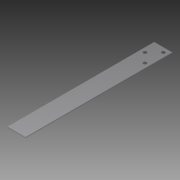
# Autodesk Inventor part: big ball holder_MIR
Saved by Autodesk Inventor 2014 SP1 (Build 180222100, 222)
## iProperties
Created: 2013-11-15
Part Number: big ball holder_MIR
Material: Polycarbonate, Clear
Document SubType Name: Modeling
Designer: RyanHughes
Density: 1.2 g/cm^3
Appearance: Polycarbonate - Clear
Author: RyanHughes
Autodesk Inventor part; units mm, degrees
ref_plane "YZ Plane" through (0, 0, 0) normal (1, 0, 0) x (0, 1, 0)
ref_plane "XZ Plane" through (0, 0, 0) normal (0, 1, 0) x (-1, 0, 0)
ref_plane "XY Plane" through (0, 0, 0) normal (0, 0, 1) x (1, 0, 0)
sketch "Sketch1" plane through (0, 0, 0) normal (0, 1, 0) x (-1, 0, 0)
  line L0 (12.7, -101.6) -> (-12.7, -101.6)
  line L1 (-12.7, -101.6) -> (-12.7, 101.6)
  line L2 (-12.7, 101.6) -> (12.7, 101.6)
  line L3 (12.7, 101.6) -> (12.7, -101.6)
  line L4 (12.7, -101.6) -> (-12.7, 101.6) construction
  line L5 (-12.7, -101.6) -> (12.7, 101.6) construction
  point P0 (0, 0)
  dimension "d0" = 25.4
  dimension "d1" = 203.2
  constraints: 12 end point, 2 midpoint, 2 parallel, 1 horizontal, 1 perpendicular
  measures "d0" distance of L1.end L2.end
  measures "d1" distance of L0.end L1.end
extrude "Extrusion1" add sketch "Sketch1" along normal blind 1.5875
sketch "Sketch2" plane through (0, 1.5875, 0) normal (0, 1, 0) x (1, 0, 0)
  line L0 (12.7, 101.6) -> (-12.7, 101.6) projected
  line L1 (-12.7, 101.6) -> (-12.7, -101.6) projected
  circle A0 centre (-6.35, 95.25) radius 2.2225
  circle A1 centre (-6.35, 82.55) radius 2.2225
  circle A2 centre (-6.35, 69.85) radius 2.2225
  circle A3 centre (6.35, 95.25) radius 2.2225
  circle A4 centre (6.35, 82.55) radius 2.2225
  circle A5 centre (6.35, 69.85) radius 2.2225
  point P0 (0, 0)
  dimension "d4" = 4.445
  dimension "d5" = 6.35
  dimension "d6" = 6.35
  dimension "d9" = 12.7
  dimension "d12" = 12.7
  constraints: 6 centre point, 1 horizontal, 1 vertical, 10 other
  measures "d4" diameter of A0
  measures "d5" distance from line of L1 A0.centre
  measures "d6" distance from line of L0 A0.centre
  measures "d9" distance of A0.centre A1.centre
  measures "d12" distance of A0.centre A3.centre
extrude "Extrusion2" cut sketch "Sketch2" against normal blind 1.5875 contours A1 | A3 | A5
fillet "Fillet1" radius 0.508 18 edges at (-12.7, 1.5875, 0) (0, 1.5875, -101.6) (0, 1.5875, 101.6) (12.7, 1.5875, 0) (-8.5725, 1.5875, -82.55) (4.1275, 1.5875, -95.25) (4.1275, 1.5875, -69.85) (4.1275, 0, -69.85) (-8.5725, 0, -82.55) (4.1275, 0, -95.25) (0, 0, -101.6) (12.7, 0, 0) (0, 0, 101.6) (-12.7, 0, 0) (12.7, 0.7937, 101.6) (-12.7, 0.7937, 101.6) (-12.7, 0.7937, -101.6) (12.7, 0.7937, -101.6)
body "Solid1"
